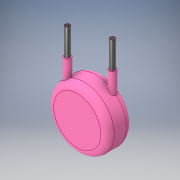
# Autodesk Inventor part: 9mm_5mm_MOV
Saved by Autodesk Inventor 2016 (Build 200138000, 138)
## iProperties
Created: 2016-09-30
Part Number: 9mm_5mm_MOV
Material: Generic
Document SubType Name: Modeling
Designer: jfixelle
Density: 1 g/cm^3
Appearance: Pink
Author: jfixelle
Autodesk Inventor part; units mm, degrees
ref_plane "YZ Plane" through (0, 0, 0) normal (1, 0, 0) x (0, 1, 0)
ref_plane "XZ Plane" through (0, 0, 0) normal (0, 1, 0) x (-1, 0, 0)
ref_plane "XY Plane" through (0, 0, 0) normal (0, 0, 1) x (1, 0, 0)
sketch "Sketch1" plane through (0, 0, 0) normal (0, 0, 1) x (1, 0, 0)
  circle A0 centre (0, 0) radius 4.5
  dimension "d0" = 9
  constraints: 1 centre point, 1 coincident
  measures "d0" diameter of A0
extrude "Extrusion1" add sketch "Sketch1" along normal mid plane 3.8
fillet "Fillet1" radius 1 2 edges at (-4.5, 0, 1.9) (-4.5, 0, -1.9)
sketch "Sketch2" plane through (0, 0, 0) normal (0, 1, 0) x (-1, 0, 0)
  circle A0 centre (-2.5, -0.85) radius 0.5
  circle A1 centre (2.5, 0.85) radius 0.5
  point P0 (0, 0)
  dimension "d4" = 2.5
  dimension "d5" = 2.5
  dimension "d8" = 1
  dimension "d9" = 1
  dimension "d12" = 0.85
  dimension "d13" = 0.85
  constraints: 2 centre point
  measures "d4" horizontal distance of point (0, 0) A0.centre
  measures "d5" horizontal distance of A1.centre point (0, 0)
  measures "d8" diameter of A1
  measures "d9" diameter of A0
  measures "d12" vertical distance of point (0, 0) A0.centre
  measures "d13" vertical distance of point (0, 0) A1.centre
extrude "Extrusion2" add sketch "Sketch2" along normal blind 6.5
sketch "Sketch3" plane through (2.5, 6.5, -0.85) normal (0, 1, 0) x (1, 0, 0)
  circle A0 centre (-5, -1.7) radius 0.35
  circle A1 centre (0, 0) radius 0.35
  point P0 (-2.5, -0.85)
  dimension "d14" = 0.85
  dimension "d15" = 0.85
  dimension "d16" = 2.5
  dimension "d17" = 2.5
  dimension "d18" = 0.7
  dimension "d19" = 0.7
  constraints: 2 centre point
  measures "d14" vertical distance of point (-2.5, -0.85) A1.centre
  measures "d15" vertical distance of point (-2.5, -0.85) A0.centre
  measures "d16" horizontal distance of point (-2.5, -0.85) A0.centre
  measures "d17" horizontal distance of A1.centre point (-2.5, -0.85)
  measures "d18" diameter of A1
  measures "d19" diameter of A0
extrude "Extrusion3" add sketch "Sketch3" along normal blind 4
body "Solid1"
